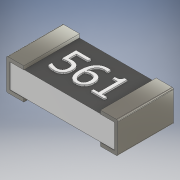
# Autodesk Inventor part: 21-1001
Saved by Autodesk Inventor 2018 (Build 220112000, 112)
## iProperties
Created: 2019-09-21
Part Number: 21-1001
Material: Copper
Document SubType Name: Modeling
Designer: Bradley
Density: 8.94 g/cm^3
Appearance: Smooth - White
Author: Bradley
Autodesk Inventor part; units mm, degrees
ref_plane "YZ Plane" through (0, 0, 0) normal (1, 0, 0) x (0, 1, 0)
ref_plane "XZ Plane" through (0, 0, 0) normal (0, 1, 0) x (-1, 0, 0)
ref_plane "XY Plane" through (0, 0, 0) normal (0, 0, 1) x (1, 0, 0)
sketch "Sketch1" plane through (0, 0, 0) normal (0, 1, 0) x (-1, 0, 0)
  line L0 (0.75, 0.175) -> (-0.75, 0.175)
  line L1 (-0.75, 0.175) -> (-0.75, -0.175)
  line L2 (-0.75, -0.175) -> (0.75, -0.175)
  line L3 (0.75, -0.175) -> (0.75, 0.175)
  line L4 (0.55, 0.175) -> (0.55, 0.225)
  line L5 (0.55, 0.225) -> (0.8, 0.225)
  line L6 (0.8, 0.225) -> (0.8, -0.225)
  line L7 (0.8, -0.225) -> (0.55, -0.225)
  line L8 (0.55, -0.225) -> (0.55, -0.175)
  line L9 (-0.55, 0.175) -> (-0.55, 0.225)
  line L10 (-0.55, 0.225) -> (-0.8, 0.225)
  line L11 (-0.8, 0.225) -> (-0.8, -0.225)
  line L12 (-0.8, -0.225) -> (-0.55, -0.225)
  line L13 (-0.55, -0.175) -> (-0.55, -0.225)
  line L14 (0.55, 0.175) -> (-0.55, 0.175)
  point P0 (0, 0)
  point P1 (0, 0.175)
  point P2 (0.75, 0)
  dimension "d0" = 1.6
  dimension "d1" = 0.05
  dimension "d2" = 0.05
  dimension "d3" = 0.45
  dimension "d4" = 0.25
  constraints: 30 end point, 12 point on line, 7 perpendicular, 3 collinear, 3 midpoint, 2 parallel, 1 horizontal, 1 horizontal alignment, 1 vertical, 1 vertical alignment
  measures "d0" distance between parallel lines of L11 L6
  measures "d1" distance of L7.end L8.end
  measures "d2" distance between parallel lines of L6 L3
  measures "d3" distance of L5.end L6.end
  measures "d4" distance of L6.end L7.end
extrude "Extrusion1" add sketch "Sketch1" along normal mid plane 0.8 contours L0 L4 L5 L6 L7 L8 L2 L3 | L0 L1 L2 L13 L12 L11 L10 L9
extrude "Extrusion2" add sketch "Sketch1" along normal mid plane 0.79 contours L3 L2 L1 L0
sketch "Sketch2" plane through (-0.55, -0.395, 0.175) normal (0, 0, 1) x (1, 0, 0)
  line L0 (0, 0) -> (0, 0.79) projected
  line L1 (1.1, 0) -> (0, 0) projected
  line L2 (1.1, 0) -> (1.1, 0.79) projected
  line L3 (0, 0.79) -> (1.1, 0.79) projected
  line L4 (0, 0.395) -> (1.1, 0.395) construction
  spline S0 degree 2 poles (0.3714, 0.3221) (0.3714, 0.2932) (0.3529, 0.2439) (0.3361, 0.2258) knots 0 0 0 1 2 2 2
  spline S1 degree 2 poles (0.3361, 0.2258) (0.3192, 0.2076) (0.269, 0.1866) (0.2378, 0.1866) knots 0 0 0 1 2 2 2
  spline S2 degree 2 poles (0.2378, 0.1866) (0.2093, 0.1866) (0.1536, 0.1992) (0.1331, 0.2093) knots 0 0 0 1 2 2 2
  line L5 (0.1331, 0.2093) -> (0.1331, 0.266)
  line L6 (0.1331, 0.266) -> (0.137, 0.266)
  spline S3 degree 2 poles (0.137, 0.266) (0.1432, 0.2615) (0.1662, 0.2498) (0.1801, 0.2446) knots 0 0 0 1 2 2 2
  spline S4 degree 2 poles (0.1801, 0.2446) (0.196, 0.2391) (0.2223, 0.2329) (0.2388, 0.2329) knots 0 0 0 1 2 2 2
  spline S5 degree 2 poles (0.2388, 0.2329) (0.255, 0.2329) (0.2855, 0.2446) (0.2965, 0.2572) knots 0 0 0 1 2 2 2
  spline S6 degree 2 poles (0.2965, 0.2572) (0.3066, 0.2692) (0.3169, 0.301) (0.3169, 0.3224) knots 0 0 0 1 2 2 2
  spline S7 degree 2 poles (0.3169, 0.3224) (0.3169, 0.3438) (0.3053, 0.371) (0.2942, 0.3801) knots 0 0 0 1 2 2 2
  spline S8 degree 2 poles (0.2942, 0.3801) (0.2829, 0.3901) (0.2492, 0.3986) (0.2288, 0.3986) knots 0 0 0 1 2 2 2
  spline S9 degree 2 poles (0.2288, 0.3986) (0.2067, 0.3986) (0.163, 0.3918) (0.1497, 0.3888) knots 0 0 0 1 2 2 2
  line L7 (0.1497, 0.3888) -> (0.1497, 0.595)
  line L8 (0.1497, 0.595) -> (0.3691, 0.595)
  line L9 (0.3691, 0.595) -> (0.3691, 0.548)
  line L10 (0.3691, 0.548) -> (0.2012, 0.548)
  line L11 (0.2012, 0.548) -> (0.2012, 0.4414)
  spline S10 degree 2 poles (0.2012, 0.4414) (0.2109, 0.4426) (0.2297, 0.4436) (0.2375, 0.4436) knots 0 0 0 1 2 2 2
  spline S11 degree 2 poles (0.2375, 0.4436) (0.2683, 0.4436) (0.3108, 0.4336) (0.3302, 0.4187) knots 0 0 0 1 2 2 2
  spline S12 degree 2 poles (0.3302, 0.4187) (0.35, 0.4038) (0.3714, 0.3584) (0.3714, 0.3221) knots 0 0 0 1 2 2 2
  spline S13 degree 2 poles (0.6819, 0.3247) (0.6819, 0.2939) (0.6615, 0.2417) (0.6443, 0.2242) knots 0 0 0 1 2 2 2
  spline S14 degree 2 poles (0.6443, 0.2242) (0.6265, 0.2057) (0.5818, 0.1866) (0.5549, 0.1866) knots 0 0 0 1 2 2 2
  spline S15 degree 2 poles (0.5549, 0.1866) (0.528, 0.1866) (0.4835, 0.2047) (0.4667, 0.2229) knots 0 0 0 1 2 2 2
  spline S16 degree 2 poles (0.4667, 0.2229) (0.4459, 0.2446) (0.4226, 0.3175) (0.4226, 0.3707) knots 0 0 0 1 2 2 2
  spline S17 degree 2 poles (0.4226, 0.3707) (0.4226, 0.4229) (0.444, 0.5068) (0.4664, 0.5379) knots 0 0 0 1 2 2 2
  spline S18 degree 2 poles (0.4664, 0.5379) (0.4881, 0.5684) (0.5568, 0.6025) (0.6019, 0.6025) knots 0 0 0 1 2 2 2
  spline S19 degree 2 poles (0.6019, 0.6025) (0.6152, 0.6025) (0.6385, 0.5999) (0.6472, 0.5969) knots 0 0 0 1 2 2 2
  line L12 (0.6472, 0.5969) -> (0.6472, 0.5454)
  line L13 (0.6472, 0.5454) -> (0.645, 0.5454)
  spline S20 degree 2 poles (0.645, 0.5454) (0.6375, 0.5493) (0.6103, 0.5561) (0.5947, 0.5561) knots 0 0 0 1 2 2 2
  spline S21 degree 2 poles (0.5947, 0.5561) (0.5448, 0.5561) (0.4835, 0.4887) (0.4777, 0.4226) knots 0 0 0 1 2 2 2
  spline S22 degree 2 poles (0.4777, 0.4226) (0.4968, 0.4358) (0.537, 0.4504) (0.561, 0.4504) knots 0 0 0 1 2 2 2
  spline S23 degree 2 poles (0.561, 0.4504) (0.5844, 0.4504) (0.6194, 0.441) (0.6385, 0.4268) knots 0 0 0 1 2 2 2
  spline S24 degree 2 poles (0.6385, 0.4268) (0.6605, 0.4102) (0.6819, 0.359) (0.6819, 0.3247) knots 0 0 0 1 2 2 2
  spline S25 degree 2 poles (0.6275, 0.3224) (0.6275, 0.347) (0.6145, 0.3804) (0.6002, 0.3921) knots 0 0 0 1 2 2 2
  spline S26 degree 2 poles (0.6002, 0.3921) (0.5895, 0.4005) (0.563, 0.406) (0.549, 0.406) knots 0 0 0 1 2 2 2
  spline S27 degree 2 poles (0.549, 0.406) (0.5302, 0.406) (0.4949, 0.3947) (0.4777, 0.384) knots 0 0 0 1 2 2 2
  spline S28 degree 2 poles (0.4777, 0.384) (0.4774, 0.3781) (0.4767, 0.3671) (0.4767, 0.3587) knots 0 0 0 1 2 2 2
  spline S29 degree 2 poles (0.4767, 0.3587) (0.4767, 0.3172) (0.4929, 0.2663) (0.5053, 0.253) knots 0 0 0 1 2 2 2
  spline S30 degree 2 poles (0.5053, 0.253) (0.5166, 0.2404) (0.5412, 0.2303) (0.5552, 0.2303) knots 0 0 0 1 2 2 2
  spline S31 degree 2 poles (0.5552, 0.2303) (0.5876, 0.2303) (0.6275, 0.2764) (0.6275, 0.3224) knots 0 0 0 1 2 2 2
  line L14 (0.9558, 0.195) -> (0.7607, 0.195)
  line L15 (0.7607, 0.195) -> (0.7607, 0.2358)
  line L16 (0.7607, 0.2358) -> (0.8333, 0.2358)
  line L17 (0.8333, 0.2358) -> (0.8333, 0.5039)
  line L18 (0.8333, 0.5039) -> (0.7607, 0.5039)
  line L19 (0.7607, 0.5039) -> (0.7607, 0.5405)
  spline S32 degree 2 poles (0.7607, 0.5405) (0.8019, 0.5405) (0.8408, 0.5639) (0.8434, 0.5963) knots 0 0 0 1 2 2 2
  line L20 (0.8434, 0.5963) -> (0.8848, 0.5963)
  line L21 (0.8848, 0.5963) -> (0.8848, 0.2358)
  line L22 (0.8848, 0.2358) -> (0.9558, 0.2358)
  line L23 (0.9558, 0.2358) -> (0.9558, 0.195)
  point P0 (0.55, 0.395)
  constraints: 2 end point, 2 midpoint, 1 horizontal
extrude "Extrusion3" add sketch "Sketch2" along normal blind 0.02 contours S0 S1 S2 L5 L6 S3 S4 S5 S6 S7 S8 S9 L7 L8 L9 L10 L11 S10 S11 S12 | S13 S14 S15 S16 S17 S18 S19 L12 L13 S20 S21 S22 S23 S24 | L14 L15 L16 L17 L18 L19 S32 L20 L21 L22 L23
fillet "Fillet1" radius 0.02 4 edges at (-0.8, 0, 0.225) (-0.8, 0, -0.225) (0.8, 0, 0.225) (0.8, 0, -0.225)
equation "\"d2\" = d1"
body "Solid1"
